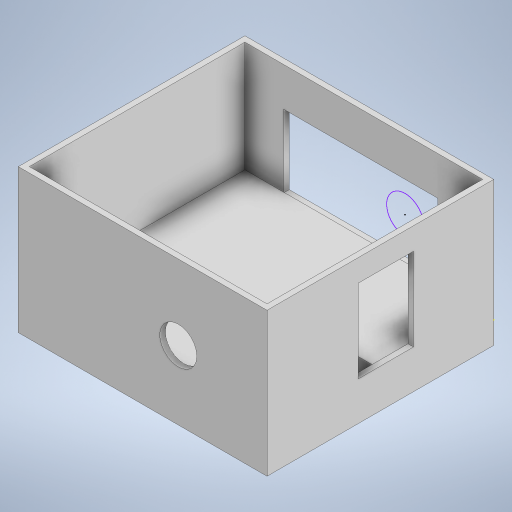
# Autodesk Inventor part: Część4
Saved by Autodesk Inventor 2024.3 (Build 283343000, 343)
## iProperties
Created: 2024-07-18
Part Number: Część4
Material: Ogólny
Document SubType Name: Modeling
Designer: User
Density: 1 g/cm^3
Appearance: Domyślna
Author: User
Autodesk Inventor part; units mm, degrees
ref_plane "YZ Plane" through (0, 0, 0) normal (1, 0, 0) x (0, 1, 0)
ref_plane "XZ Plane" through (0, 0, 0) normal (0, 1, 0) x (-1, 0, 0)
ref_plane "XY Plane" through (0, 0, 0) normal (0, 0, 1) x (1, 0, 0)
sketch "Szkic1" plane through (0, 0, 0) normal (0, 1, 0) x (-1, 0, 0)
  line L0 (0, 0) -> (45, 0)
  line L1 (45, 0) -> (45, -41)
  line L2 (45, -41) -> (0, -41)
  line L3 (0, -41) -> (0, 0)
  line L4 (45, 0) -> (44, 0)
  line L5 (44, 0) -> (44, -1)
  line L6 (0, -41) -> (0, -40)
  line L7 (0, -40) -> (1, -40)
  line L8 (1, -40) -> (44, -40)
  line L9 (44, -40) -> (44, -1)
  line L10 (44, -1) -> (1, -1)
  line L11 (1, -1) -> (1, -40)
  dimension "d0" = 45
  dimension "d1" = 41
  dimension "d2" = 1
  dimension "d3" = 1
  dimension "d4" = 1
  dimension "d5" = 1
  constraints: 24 end point, 4 parallel, 4 perpendicular, 2 horizontal, 2 point on line
  measures "d0" distance of L1.end L2.end
  measures "d1" distance of L0.end L1.end
  measures "d2" distance of L0.end L4.end
  measures "d3" distance of L4.end L5.end
  measures "d4" distance of L2.end L6.end
  measures "d5" distance of L6.end L7.end
extrude "Wyciągnięcie proste1" add sketch "Szkic1" along normal blind 18 contours L0 L5 L10 L11 L7 L3 | L0 L1 L2 L3 L7 L8 L9 L5
sketch "Szkic2" plane through (0, 0, -41) normal (0, 0, -1) x (-1, 0, 0)
  line L0 (40, 15) -> (12.1, 15)
  line L1 (12.1, 15) -> (12.1, 1.9)
  line L2 (12.1, 1.9) -> (40, 1.9)
  line L3 (40, 1.9) -> (40, 15)
  line L4 (40, 8.45) -> (38, 8.45)
  line L5 (12.1, 8.45) -> (10.1, 8.45)
  line L6 (10.1, 8.45) -> (38, 8.45)
  line L7 (38, 8.45) -> (38, 15)
  line L8 (38, 15) -> (10.1, 15)
  line L9 (10.1, 15) -> (10.1, 8.45)
  line L10 (38, 8.45) -> (10.1, 8.45)
  line L11 (10.1, 8.45) -> (10.1, 1.9)
  line L12 (10.1, 1.9) -> (38, 1.9)
  line L13 (38, 1.9) -> (38, 8.45)
  line L14 (10.1, 1.9) -> (9.1, 1.9)
  line L15 (9.1, 1.9) -> (9.1, 15)
  line L16 (9.1, 15) -> (10.1, 15)
  line L17 (10.1, 15) -> (10.1, 1.9)
  line L18 (38, 1.9) -> (37, 1.9)
  line L19 (37, 1.9) -> (37, 15)
  line L20 (37, 15) -> (38, 15)
  line L21 (38, 15) -> (38, 1.9)
  point P0 (0, 0)
  point P1 (10.1, 15)
  dimension "d8" = 27.9
  dimension "d9" = 13.1
  dimension "d33" = 2
  dimension "d34" = 2
  dimension "d35" = 1
  dimension "d36" = 1
  constraints: 44 end point, 10 parallel, 7 horizontal, 5 perpendicular, 3 point on line, 2 midpoint
  measures "d8" distance of L2.end L1.end
  measures "d9" distance of L1.end L0.end
  measures "d33" distance of L4.start L4.end
  measures "d34" distance of L5.start L5.end
  measures "d35" distance of L15.end L16.end
  measures "d36" distance of L19.end L20.end
extrude "Wyciągnięcie proste2" cut sketch "Szkic2" against normal blind 5.25 contours L19 L6 L1 L0 | L1 L5 L9 L8 | L19 L2 L1 L6 | L1 L12 L11 L5 | L9 L11 L14 L15 L16
sketch "Szkic3" plane through (0, 0, -41) normal (0, 0, -1) x (-1, 0, 0)
  line L0 (12.1, 1.9) -> (12.1, 15) projected
  line L1 (12.1, 8.45) -> (21.9, 8.45)
  line L2 (21.9, 8.45) -> (19.05, 8.45)
  circle A0 centre (19.05, 8.45) radius 3.35
  line L3 (19.05, 8.45) -> (16.05, 8.45)
  circle A1 centre (16.05, 8.45) radius 3.35
  point P0 (0, 0)
  dimension "d12" = 9.8
  dimension "d13" = 2.85
  dimension "d14" = 6.7
  dimension "d37" = 3
  dimension "d38" = 6.7
  constraints: 6 end point, 2 centre point, 2 coincident, 2 point on line, 1 horizontal, 1 midpoint
  measures "d12" distance of L1.start L1.end
  measures "d13" distance of L1.end L2.end
  measures "d14" diameter of A0
  measures "d37" distance of L3.start L3.end
  measures "d38" diameter of A1
extrude "Wyciągnięcie proste3" cut sketch "Szkic3" against normal blind 48.25 contours L1 A0 A1 | L1 A1 A0 | A0 A1 L1 | L1 A1 A0
sketch "Szkic4" plane through (0, 0, 0) normal (1, 0, 0) x (0, 0, -1)
  line L0 (1, 18) -> (40, 18) projected
  line L1 (20.5, 18) -> (26.5, 18)
  line L2 (26.5, 18) -> (26.5, 3)
  line L3 (26.5, 3) -> (20.5, 3)
  line L4 (20.5, 3) -> (20.5, 18)
  line L5 (20.5, 18) -> (16.5, 18)
  line L6 (16.5, 18) -> (16.5, 3)
  line L7 (16.5, 3) -> (20.5, 3)
  line L8 (20.5, 3) -> (20.5, 18)
  point P0 (0, 0)
  dimension "d17" = 6
  dimension "d18" = 15
  dimension "d19" = 4
  constraints: 16 end point, 4 parallel, 2 horizontal, 2 perpendicular, 1 midpoint, 1 point on line
  measures "d17" distance of L2.end L3.end
  measures "d18" distance of L1.end L2.end
  measures "d19" distance of L7.end L6.end
extrude "Wyciągnięcie proste4" cut sketch "Szkic4" against normal blind 24.25
sketch "Szkic5" plane through (0, 0, 0) normal (0, -1, 0) x (1, 0, 0)
  line L0 (-1, -40) -> (-1, -26.5) projected
  line L1 (-44, -1) -> (-44, -40) projected
  line L2 (-1, -40) -> (-44, -40)
  line L3 (-44, -40) -> (-44, -21)
  line L4 (-44, -21) -> (-1, -21)
  line L5 (-1, -21) -> (-1, -40)
  line L6 (0, 0) -> (0, -41) projected
  line L7 (0, -41) -> (-45, -41) projected
  line L8 (0, -21) -> (-45, -21)
  line L9 (-45, -21) -> (-45, -41)
  line L10 (-45, -41) -> (0, -41)
  line L11 (0, -41) -> (0, -21)
  dimension "d22" = 19
  constraints: 16 end point, 4 parallel, 3 point on line, 2 horizontal, 2 perpendicular
  measures "d22" distance of L2.end L3.end
extrude "Wyciągnięcie proste5" add sketch "Szkic5" against normal blind 2 contours L2 L1 L4 L5 L0
sketch "Szkic6" plane through (0, 0, 0) normal (0, -1, 0) x (1, 0, 0)
  line L0 (0, 0) -> (-45, 0)
  line L1 (-45, 0) -> (-45, -40.9786)
  line L2 (-45, -40.9786) -> (0, -40.9786)
  line L3 (0, -40.9786) -> (0, 0)
  constraints: 8 end point, 2 parallel, 1 horizontal, 1 perpendicular
extrude "Wyciągnięcie proste6" add sketch "Szkic6" along normal blind 4
sketch "Szkic7" plane through (0, 0, 0) normal (0, 1, 0) x (1, 0, 0)
  line L0 (-1, 1) -> (-44, 1) projected
  line L1 (-44, 21) -> (-1, 21) projected
  line L2 (-44, 1) -> (-1, 1)
  line L3 (-1, 1) -> (-1, 21)
  line L4 (-1, 21) -> (-44, 21)
  line L5 (-44, 21) -> (-44, 1)
  point P0 (0, 0)
  constraints: 8 end point, 2 parallel, 1 horizontal, 1 perpendicular
extrude "Wyciągnięcie proste7" cut sketch "Szkic7" against normal blind 2
sketch "Szkic8" plane through (0, 0, -40.9786) normal (0, 0, -1) x (-1, 0, 0)
  line L0 (45, -4) -> (0, -4) projected
  line L1 (0, 0) -> (45, 0) projected
  line L2 (45, -4) -> (0, -4)
  line L3 (0, -4) -> (0, 0)
  line L4 (0, 0) -> (45, 0)
  line L5 (45, 0) -> (45, -4)
  constraints: 8 end point, 2 parallel, 1 horizontal, 1 perpendicular
extrude "Wyciągnięcie proste8" add sketch "Szkic8" along normal blind 0.0214
sketch "Szkic9" plane through (0, 18, 0) normal (0, 1, 0) x (1, 0, 0)
  line L0 (0, 26.5) -> (0, 41) projected
  line L1 (0, 0) -> (-45, 0) projected
  line L2 (0, 41) -> (-45, 41)
  line L3 (-45, 41) -> (-45, 0)
  line L4 (-45, 0) -> (0, 0)
  line L5 (0, 0) -> (0, 41)
  line L6 (-1, 40) -> (-1, 26.5) projected
  line L7 (-44, 1) -> (-44, 40) projected
  line L8 (-1, 40) -> (-44, 40)
  line L9 (-44, 40) -> (-44, 1)
  line L10 (-44, 1) -> (-1, 1)
  line L11 (-1, 1) -> (-1, 40)
  constraints: 16 end point, 4 parallel, 2 horizontal, 2 perpendicular
extrude "Wyciągnięcie proste9" add sketch "Szkic9" along normal blind 4
sketch "Szkic10" plane through (0, -4, -41) normal (0, 0, -1) x (-1, 0, 0)
  circle A0 centre (16.05, 12.45) radius 3.35 projected
  circle A1 centre (16.05, 12.45) radius 3.35
  point P0 (0, 4)
  constraints: 1 centre point, 1 coincident
